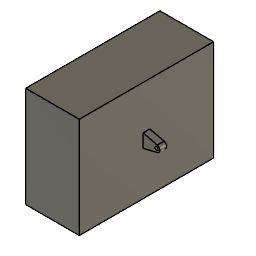
headlike_robotic_eye_assembly (Autodesk Fusion 360 archive; units mm, degrees)
design "Linear Actuator"
Autodesk Fusion 360 part; units mm, degrees
sketch "草图1" plane through (0, 0, 0) normal (1, 0, 0) x (0, 1, 0)
  line L0 (10, 7.5) -> (-10, 7.5)
  line L1 (-10, 7.5) -> (-10, -7.5)
  line L2 (-10, -7.5) -> (10, -7.5)
  line L3 (10, -7.5) -> (10, 7.5)
  line L4 (10, 7.5) -> (-10, -7.5) construction
  line L5 (-10, 7.5) -> (10, -7.5) construction
  dimension "d1" = 20
  dimension "d2" = 15
  constraint horizontal L0
  constraint perpendicular L0 L1
  constraint parallel L0 L2
  constraint parallel L1 L3
  constraint coincident L4 origin
  constraint coincident L5 origin
  measures "d1" distance of L1.end L2.end
  measures "d2" distance of L0.end L1.end
extrude "拉伸1" add sketch "草图1" along normal mid plane 8
sketch "草图2" plane through (0, 0, 0) normal (0, 1, 0) x (1, 0, 0)
  line L0 (4, 0) -> (4, 1)
  line L1 (4, 0) -> (4, -1)
  circle A0 centre (6, 0) radius 0.5
  line L2 (4, 7.5) -> (4, -7.5)
  line L3 (4, 1) -> (6.1179, 0.4859)
  line L4 (4, -1) -> (6.1179, -0.4859)
  circle A1 centre (6, 0) radius 0.25
  dimension "d5" = 1
  dimension "d6" = 1
  dimension "d7" = 1
  dimension "d8" = 2
  dimension "d9" = 0.5
  constraint vertical L0
  constraint parallel L0 L1
  constraint coincident A0 L3.end
  constraint tangent A0 L3
  constraint coincident A0 L4.end
  constraint tangent A0 L4
  constraint concentric A0 A1
  measures "d5" distance of L0.start L0.end
  measures "d6" distance of L0.start L1.end
  measures "d7" diameter of A0
  measures "d8" distance of A0.centre L2
  measures "d9" diameter of A1
extrude "拉伸2" add sketch "草图2" along normal mid plane 1

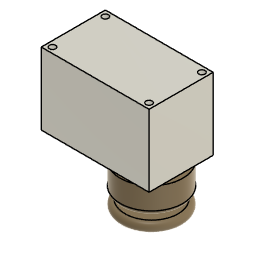
design "Robotis servo"
Autodesk Fusion 360 part; units mm, degrees
sketch "草图1" plane through (0, 0, 0) normal (0, 0, 1) x (1, 0, 0)
  line L0 (17.25, 10.25) -> (-17.25, 10.25)
  line L1 (-17.25, 10.25) -> (-17.25, -10.25)
  line L2 (-17.25, -10.25) -> (17.25, -10.25)
  line L3 (17.25, -10.25) -> (17.25, 10.25)
  line L4 (17.25, 10.25) -> (-17.25, -10.25) construction
  line L5 (-17.25, 10.25) -> (17.25, -10.25) construction
  dimension "d1" = 34.5
  dimension "d2" = 20.5
  constraint horizontal L0
  constraint perpendicular L0 L1
  constraint parallel L0 L2
  constraint parallel L1 L3
  constraint coincident L4 origin
  constraint coincident L5 origin
  measures "d1" distance of L1.end L2.end
  measures "d2" distance of L0.end L1.end
extrude "拉伸1" add sketch "草图1" along normal blind 23 makes body 1
sketch "草图2" plane through (0, 0, 0) normal (0, 0, 1) x (1, 0, 0)
  circle A0 centre (7.75, 0.0343) radius 8
  line L0 (17.25, -10.25) -> (17.25, 10.25)
  dimension "d5" = 16
  dimension "d6" = 9.5
  measures "d5" diameter of A0
  measures "d6" distance of A0.centre L0
extrude "拉伸2" add sketch "草图2" against normal blind 3 bodies 1
sketch "草图3" plane through (0, 0, -3) normal (0, 0, -1) x (1, 0, 0)
  circle A0 centre (7.75, -0.0343) radius 8
  circle A1 centre (7.75, -0.0343) radius 6
  circle A2 centre (13.75, -0.0342) radius 1.15
  circle A3 centre (7.7499, 5.9657) radius 1.15
  circle A4 centre (1.75, -0.0344) radius 1.15
  circle A5 centre (7.7501, -6.0343) radius 1.15
  dimension "d9" = 12
  dimension "d10" = 2.3
  dimension "d12" = 360
  constraint concentric A0 A1
  constraint coincident A1 A2.centre
  measures "d9" diameter of A1
  measures "d10" diameter of A2
extrude "拉伸3" cut sketch "草图3" against normal blind 3 contours A1 A2 | A1 A2 | A1 A3 | A1 A3 | A1 A5 | A1 A5 | A1 A4 | A1 A4 bodies 1
sketch "草图4" plane through (0, 0, -3) normal (0, 0, -1) x (1, 0, 0)
  circle A0 centre (1.75, -0.0344) radius 1.15
  circle A1 centre (7.7501, -6.0343) radius 1.15
  circle A2 centre (7.7499, 5.9657) radius 1.15
  circle A3 centre (13.75, -0.0342) radius 1.15
  circle A4 centre (7.75, -0.0343) radius 8
  circle A5 centre (7.75, -0.0343) radius 10
  dimension "d15" = 20
  constraint concentric A4 A5
  measures "d15" diameter of A5
extrude "拉伸4" add sketch "草图4" against normal blind 2 separate body contours A5 makes body 2
sketch "草图5" plane through (0, 0, -3) normal (0, 0, -1) x (1, 0, 0)
  circle A0 centre (1.75, -0.0344) radius 1.15
  circle A1 centre (7.7501, -6.0343) radius 1.15
  circle A2 centre (7.7499, 5.9657) radius 1.15
  circle A3 centre (13.75, -0.0342) radius 1.15
  circle A4 centre (7.75, -0.0343) radius 8
  circle A5 centre (7.75, -0.0343) radius 10
  dimension "d18" = 20
  constraint concentric A4 A5
  measures "d18" diameter of A5
extrude "拉伸5" add sketch "草图5" along normal blind 6.5 contours A4 | A5 bodies 2
sketch "草图8" plane through (0, 0, -9.5) normal (0, 0, -1) x (1, 0, 0)
  circle A0 centre (13.75, -0.0342) radius 1.15
  circle A1 centre (7.7499, 5.9657) radius 1.15
  circle A2 centre (7.7501, -6.0343) radius 1.15
  circle A3 centre (1.75, -0.0344) radius 1.15
  circle A4 centre (7.75, -0.0343) radius 10
  circle A5 centre (7.75, -0.0343) radius 6
  circle A6 centre (13.75, -0.0342) radius 2
  circle A7 centre (7.7499, 5.9657) radius 2
  circle A8 centre (1.75, -0.0344) radius 2
  circle A9 centre (7.7501, -6.0343) radius 2
  dimension "d31" = 12
  dimension "d32" = 4
  dimension "d34" = 360
  constraint concentric A4 A5
  constraint concentric A0 A6
  measures "d31" diameter of A5
  measures "d32" diameter of A6
extrude "拉伸8" cut sketch "草图8" against normal blind 1.6 contours A0 A5 A6 | A0 A5 A6 | A1 A5 A7 | A1 A5 A7 | A2 A5 A9 | A2 A5 A9 | A3 A5 A8 | A3 A5 A8 bodies 2
sketch "草图6" plane through (0, 0, -9.5) normal (0, 0, -1) x (1, 0, 0)
  circle A0 centre (7.75, -0.0343) radius 10
  circle A1 centre (7.75, -0.0343) radius 2.5
  circle A2 centre (7.7499, 5.9657) radius 2
  circle A3 centre (1.75, -0.0344) radius 2
  circle A4 centre (13.75, -0.0342) radius 2
  circle A5 centre (7.7501, -6.0343) radius 2
  dimension "d21" = 5
  constraint concentric A0 A1
  measures "d21" diameter of A1
extrude "拉伸6" add sketch "草图6" along normal blind 1.5 contours A1 bodies 2
sketch "草图7" plane through (0, 0, -11) normal (0, 0, -1) x (1, 0, 0)
  circle A0 centre (7.75, -0.0343) radius 2.5
  circle A1 centre (7.75, -0.0343) radius 10
  circle A2 centre (7.75, -0.0343) radius 6
  dimension "d24" = 20
  dimension "d27" = 12
  constraint concentric A0 A1
  constraint concentric A0 A2
  measures "d24" diameter of A1
  measures "d27" diameter of A2
extrude "拉伸7" add sketch "草图7" along normal blind 3 contours A0 | A1 | A2 bodies 2
sketch "草图9" plane through (0, 0, 23) normal (0, 0, 1) x (-1, 0, 0)
  line L0 (-17.25, 10.25) -> (-17.25, -10.25)
  line L1 (-17.25, -10.25) -> (17.25, -10.25)
  line L2 (17.25, -10.25) -> (17.25, 10.25)
  line L3 (17.25, 10.25) -> (-17.25, 10.25)
  circle A0 centre (-15.45, -8.45) radius 1
  line L4 (-20, 0) -> (-2.5, 0)
  circle A1 centre (-15.45, 8.45) radius 1
  line L5 (0, -2.5) -> (0, -20)
  circle A2 centre (15.45, 8.45) radius 1
  circle A3 centre (15.45, -8.45) radius 1
  dimension "d37" = 2
  dimension "d38" = 1.8
  dimension "d39" = 1.8
  constraint symmetric A0 L4 A1
  constraint symmetric A0 L5 A3
  constraint symmetric A1 L5 A2
  measures "d37" diameter of A0
  measures "d38" distance of L0 A0.centre
  measures "d39" distance of L1 A0.centre
extrude "拉伸9" cut sketch "草图9" against normal up to surface (23 mm away) contours A0 | A1 | A2 | A3 bodies 1
fillet "圆角1" radius 1.5 2 edges at (-1.5733, 3.6505, -9.5) (-1.5733, 3.6505, -11) on bodies 2
fillet "圆角1" radius 1.5 1 edges at (-1.5733, 3.6505, -14) on bodies 2
split "分割1" by plane through (0, 0, -9.5) normal (0, 0, -1) bodies 2 makes body 3 at (6.8779, -2.2646, -14)
extrude "拉伸10" add 1 faces at (7.6145, -0.5593, -9.5) along direction (0, 0, 1) blind 4 on bodies 3 bodies 3
extrude "拉伸11" cut 1 faces at (7.6145, -0.5593, -5.5) along direction (0, 0, 1) blind -4 and the other way blind -1 on bodies 3 bodies 2
fillet "圆角2" radius 0.5 1 edges at (5.4192, -0.8697, -9.5) on bodies 2
sketch "草图10" plane through (0, 0, -11) normal (0, 0, 1) x (-1, 0, 0)
  circle A0 centre (-7.75, -0.0343) radius 2.5
  circle A1 centre (-7.75, -0.0343) radius 8.5
  circle A2 centre (-7.75, -0.0343) radius 7.85
  dimension "d52" = 15.7
  constraint concentric A0 A2
  measures "d52" diameter of A2
extrude "拉伸12" add sketch "草图10" along normal blind 0.2 contours A2 bodies 3
sketch "草图11" plane through (0, 0, -10.8) normal (0, 0, 1) x (-1, 0, 0)
  circle A0 centre (-7.75, -0.0343) radius 2.5
  circle A1 centre (-7.75, -0.0343) radius 7.85
  circle A2 centre (-7.75, -0.0343) radius 7.5
  dimension "d55" = 15
  constraint concentric A0 A2
  measures "d55" diameter of A2
extrude "拉伸13" add sketch "草图11" along normal blind 1.7 contours A2 bodies 3
sketch "草图12" plane through (0, 0, -9.1) normal (0, 0, 1) x (-1, 0, 0)
  circle A0 centre (-7.75, -0.0343) radius 2.5
  circle A1 centre (-7.75, -0.0343) radius 7.5
  circle A2 centre (-7.75, -0.0343) radius 7.85
  dimension "d58" = 15.7
  constraint concentric A0 A2
  measures "d58" diameter of A2
extrude "拉伸14" add sketch "草图12" along normal blind 0.2 contours A1 | A2 bodies 3
fillet "圆角3" radius 1.2 2 edges at (14.7425, 2.7464, -9.1) (14.7425, -2.6778, -10.8) on bodies 3
fillet "圆角4" radius 0.7 1 edges at (5.4192, -0.8697, -5.5) on bodies 3
move_body "移动1" bodies 3 to x (1, 0, 0) y (0, 1, 0) z (0, 0, 1) at (0, 0, -4)
move_body "移动2" bodies 3 to x (1, 0, 0) y (0, 1, 0) z (0, 0, 1) at (0, 0, 3.4)
extrude "拉伸15" cut 1 faces at (1.7219, 0.5485, -9.5) along direction (0, 0, -1) up to surface (2.1 mm away) on bodies 3 bodies 3
named bodies: "servo spool 1", "servo spool 2"
